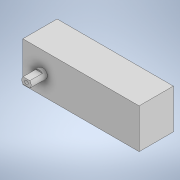
# Autodesk Inventor part: motor_placeholder
Saved by Autodesk Inventor 2021 (Build 250183000, 183)
## iProperties
Created: 2023-05-05
Part Number: motor_placeholder
Material: Generic
Document SubType Name: Modeling
Designer: assman
Density: 1 g/cm^3
Appearance: Default
Author: assman
Autodesk Inventor part; units mm, degrees
ref_plane "YZ Plane" through (0, 0, 0) normal (1, 0, 0) x (0, 1, 0)
ref_plane "XZ Plane" through (0, 0, 0) normal (0, 1, 0) x (-1, 0, 0)
ref_plane "XY Plane" through (0, 0, 0) normal (0, 0, 1) x (1, 0, 0)
sketch "Sketch1" plane through (0, 0, 0) normal (0, 1, 0) x (-1, 0, 0)
  line L0 (32.25, 9.5) -> (-32.25, 9.5)
  line L1 (-32.25, 9.5) -> (-32.25, -9.5)
  line L2 (-32.25, -9.5) -> (32.25, -9.5)
  line L3 (32.25, -9.5) -> (32.25, 9.5)
  line L4 (32.25, 9.5) -> (-32.25, -9.5) construction
  line L5 (-32.25, 9.5) -> (32.25, -9.5) construction
  point P0 (0, 0)
  dimension "d0" = 19
  dimension "d1" = 64.5
  constraints: 12 end point, 2 midpoint, 2 parallel, 1 horizontal, 1 perpendicular
  measures "d0" distance of L1.end L0.end
  measures "d1" distance of L1.end L2.end
extrude "Extrusion1" add sketch "Sketch1" along normal blind 22
sketch "Sketch2" plane through (-32.25, 0, 9.5) normal (0, 0, 1) x (1, 0, 0)
  line L0 (0, 0) -> (64.5, 0) construction
  line L1 (64.5, 0) -> (64.5, 22) construction
  line L2 (0, 22) -> (64.5, 22) construction
  line L3 (0, 0) -> (0, 22) construction
  line L4 (0, 22) -> (13.267, 8.733) construction
  line L5 (0, 22) -> (18.7624, 22) construction
  line L6 (13.267, 8.733) -> (22, 0) construction
  line L7 (64.5, 0) -> (0, 0) construction
  line L8 (0, 0) -> (22, 22) construction
  circle A0 centre (11, 11) radius 2.6
  point P0 (32.25, 0)
  dimension "d4" = 45
  dimension "d5" = 5.2
  constraints: 8 end point, 3 point on line, 1 centre point, 1 equal length, 1 horizontal, 1 midpoint
  measures "d4" angle of L4 L5
  measures "d5" diameter of A0
extrude "Extrusion2" add sketch "Sketch2" along normal blind 9
sketch "Sketch3" plane through (-21.25, 11, 18.5) normal (0, 0, 1) x (1, 0, 0)
  line L0 (-1.8762, 1.8) -> (1.8762, 1.8)
  line L1 (1.8762, -1.8) -> (-1.8762, -1.8)
  line L2 (-2.2795, 1.2506) -> (2.2795, -1.2506) construction
  line L3 (2.2795, 1.2506) -> (-2.2795, -1.2506) construction
  arc A0 (1.8762, 1.8) -> (-1.8762, 1.8) centre (0, 0) ccw
  arc A1 (-1.8762, -1.8) -> (1.8762, -1.8) centre (0, 0) ccw
  point P0 (21.25, -11)
  constraints: 8 end point, 4 point on circle, 2 centre point, 2 coincident, 2 midpoint, 1 horizontal, 1 parallel
extrude "Extrusion3" cut sketch "Sketch3" against normal blind 7
sketch "Sketch4" plane through (-32.25, 0, 18.5) normal (0, 0, 1) x (1, 0, 0)
  line L0 (9.1238, 9.2) -> (12.8762, 9.2) construction
  arc A0 (12.8762, 9.2) -> (12.8762, 12.8) centre (11, 11) ccw construction
  line L1 (12.8762, 12.8) -> (9.1238, 12.8) construction
  arc A1 (9.1238, 12.8) -> (9.1238, 9.2) centre (11, 11) ccw construction
  circle A2 centre (11, 11) radius 1
  point P0 (32.25, 0)
  dimension "d11" = 2
  constraints: 1 centre point, 1 coincident
  measures "d11" diameter of A2
extrude "Extrusion4" cut sketch "Sketch4" against normal blind 7
body "Solid1"
